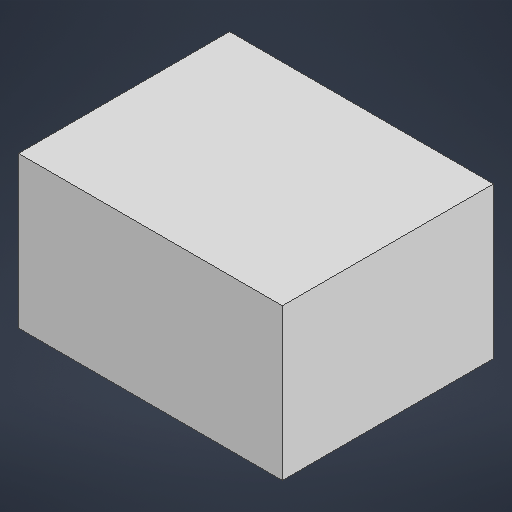
# Autodesk Inventor part: Stand of Shooting
Saved by Autodesk Inventor 2026.2 (Build 302298010, 298A)
## iProperties
Created: 2026-04-30
Part Number: Stand of Shooting
Material: Generic
Document SubType Name: Modeling
Designer: lenovo
Density: 1 g/cm^3
Appearance: Default
Author: lenovo
Autodesk Inventor part; units mm, degrees
ref_plane "YZ Plane" through (0, 0, 0) normal (1, 0, 0) x (0, 1, 0)
ref_plane "XZ Plane" through (0, 0, 0) normal (0, 1, 0) x (-1, 0, 0)
ref_plane "XY Plane" through (0, 0, 0) normal (0, 0, 1) x (1, 0, 0)
sketch "Sketch1" plane through (0, 0, 0) normal (0, 1, 0) x (-1, 0, 0)
  line L0 (-75, 60) -> (75, 60)
  line L1 (75, 60) -> (75, -60)
  line L2 (75, -60) -> (-75, -60)
  line L3 (-75, -60) -> (-75, 60)
  line L4 (-75, 60) -> (75, -60) construction
  line L5 (75, 60) -> (-75, -60) construction
  line L6 (-70, 55) -> (70, 55)
  line L7 (70, 55) -> (70, -55)
  line L8 (70, -55) -> (-70, -55)
  line L9 (-70, -55) -> (-70, 55)
  line L10 (-70, 55) -> (70, -55) construction
  line L11 (70, 55) -> (-70, -55) construction
  point P0 (0, 0)
  dimension "d0" = 150
  dimension "d1" = 120
  dimension "d2" = 140
  dimension "d3" = 110
  dimension "d8" = 5
  constraints: 24 end point, 4 midpoint, 4 parallel, 2 horizontal, 2 perpendicular
  measures "d0" distance of L1.end L2.end
  measures "d1" distance of L0.end L1.end
  measures "d2" distance of L7.end L8.end
  measures "d3" distance of L6.end L7.end
  measures "d8" distance between parallel lines of L3 L9
extrude "Extrusion1" add sketch "Sketch1" along normal blind 86 contours L0 L1 L2 L3 | L6 L7 L8 L9
extrude "Extrusion2" cut sketch "Sketch1" along normal blind 81 contours L6 L7 L8 L9
body "Solid1"
